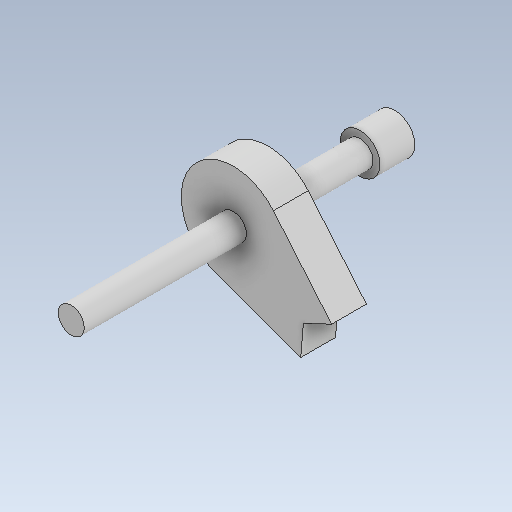
# Autodesk Inventor part: reverser-base
Saved by Autodesk Inventor 2021 (Build 250183000, 183)
## iProperties
Created: 2021-07-09
Part Number: reverser-base
Material: Generic
Document SubType Name: Modeling
Designer: teh18
Density: 1 g/cm^3
Appearance: Default
Author: teh18
Autodesk Inventor part; units mm, degrees
ref_plane "YZ Plane" through (0, 0, 0) normal (1, 0, 0) x (0, 1, 0)
ref_plane "XZ Plane" through (0, 0, 0) normal (0, 1, 0) x (-1, 0, 0)
ref_plane "XY Plane" through (0, 0, 0) normal (0, 0, 1) x (1, 0, 0)
sketch "Sketch1" plane through (0, 0, 0) normal (0, 0, 1) x (1, 0, 0)
  line L0 (3, -1) -> (-3, -1) projected
  line L1 (-3, -1) -> (-3, 1) projected
  line L2 (-3, 1) -> (3, 1) projected
  line L3 (3, 1) -> (3, -1) projected
  circle A0 centre (0, 0) radius 3.75 projected
  line L4 (-3.1, 1.1) -> (-3.1, -1.1)
  line L5 (-3.1, -1.1) -> (3.1, -1.1)
  line L6 (3.1, -1.1) -> (3.1, 1.1)
  line L7 (3.1, 1.1) -> (-3.1, 1.1)
  circle A1 centre (0, 0) radius 5.75
  dimension "d0" = 0.1
  dimension "d5" = 2
  constraints: 8 end point, 1 centre point, 3 other
  measures "d0" distance between parallel lines of L1 L4
  measures "d5" radial gap between concentric circles of A0 A1
extrude "Extrusion1" add sketch "Sketch1" along normal blind 10 contours A0 | A1
sketch "Sketch2" plane through (0, 0, 10) normal (0, 0, 1) x (0, -1, 0)
  line L0 (-1.1, -3.1) -> (-1.1, 3.1) projected
  line L1 (-1.1, 3.1) -> (1.1, 3.1) projected
  line L2 (1.1, 3.1) -> (1.1, -3.1) projected
  line L3 (1.1, -3.1) -> (-1.1, -3.1) projected
  circle A0 centre (0, 0) radius 3.75
  constraints: 1 centre point, 2 other
ref_plane "Work Plane1" through (-14, -11, 93) normal (0, 0, -1) x (0, 1, 0)
extrude "Extrusion2" add sketch "Sketch2" along normal up to surface (83 mm away) contours L0 L1 L2 L3 | A0
ref_plane "Work Plane2" through (0, 0, 36.375) normal (0, 0, -1) x (-1, 0, 0)
sketch "Sketch3" plane through (0, 0, 36.375) normal (0, 0, -1) x (-1, 0, 0)
  circle A0 centre (0, 0) radius 15
  arc A1 (-91.9148, -71.9535) -> (-91.7708, -72.0943) centre (-67.3725, -47) ccw projected
  arc A2 (-99.8859, -53.9357) -> (-101.7483, -40.4192) centre (-102.3703, -47.3915) ccw projected
  arc A3 (-60.0244, -81.22) -> (-73.5792, -79.6604) centre (-66.981, -81.9978) ccw projected
  circle A4 centre (0, 0) radius 30
  line L0 (0, 0) -> (-28.2086, -10.2115)
  line L1 (0, 0) -> (30, 0) construction
  line L2 (0, 0) -> (-19.3236, -22.9477)
  line L3 (0, 0) -> (30, 0) construction
  line L4 (0, 0) -> (-20.0895, -14.0147)
  line L5 (0, 0) -> (25, 0) construction
  line L6 (-19.3236, -22.9477) -> (-20.0895, -14.0147)
  line L7 (-20.0895, -14.0147) -> (-28.2086, -10.2115)
  line L8 (-19.3236, -22.9477) -> (5.1057, -14.1043)
  line L9 (-28.2086, -10.2115) -> (-11.4738, 9.6618)
  arc A5 (-75.9549, -80.9315) -> (-73.5792, -79.6604) centre (-75.4644, -78.9925) ccw projected
  arc A6 (-60.0244, -81.22) -> (-56.998, -80.4271) centre (-67.3725, -47) ccw projected
  line L10 (-56.998, -80.4271) -> (-59.9621, -70.8765) projected
  arc A7 (-59.9621, -70.8765) -> (-52.3252, -27.0356) centre (-67.3725, -47) ccw projected
  line L11 (-52.3252, -27.0356) -> (-43.825, -21.1057) projected
  arc A8 (-76.15, -80.8815) -> (-75.9549, -80.9315) centre (-67.3725, -47) ccw projected
  arc A9 (-99.8859, -53.9357) -> (-101.1035, -56.3392) centre (-99.176, -55.8055) ccw projected
  arc A10 (-101.0492, -56.5332) -> (-98.7606, -57.955) centre (-99.1248, -55.9884) ccw projected
  arc A11 (-92.062, -69.2632) -> (-98.7606, -57.955) centre (-97.4858, -64.8379) ccw projected
  arc A12 (-92.062, -69.2632) -> (-91.9148, -71.9535) centre (-90.5124, -70.5276) ccw projected
  arc A13 (-91.7708, -72.0943) -> (-89.0779, -72.1813) centre (-90.3766, -70.6604) ccw projected
  arc A14 (-77.6226, -78.6253) -> (-89.0779, -72.1813) centre (-84.5324, -77.5047) ccw projected
  arc A15 (-77.6226, -78.6253) -> (-76.15, -80.8815) centre (-75.6484, -78.9454) ccw projected
  circle A16 centre (-67.3725, -47) radius 18 projected
  circle A17 centre (-67.3725, -47) radius 18 projected
  line L12 (-87.3977, -18.2947) -> (-93.1192, -10.0932) projected
  arc A18 (-93.1192, -10.0932) -> (-111.0378, -36.1215) centre (-67.3725, -47) ccw projected
  line L13 (-111.0378, -36.1215) -> (-101.3344, -38.5389) projected
  arc A19 (-101.3344, -38.5389) -> (-101.7483, -40.4192) centre (-67.3725, -47) ccw projected
  arc A20 (-43.825, -21.1057) -> (-87.3977, -18.2947) centre (-67.3725, -47) ccw projected
  arc A21 (-101.1035, -56.3392) -> (-101.0492, -56.5332) centre (-67.3725, -47) ccw projected
  point P0 (-85.3708, -47.2511)
  point P1 (-67.1214, -64.9982)
  point P2 (-67.3725, -47)
  point P3 (-99.176, -55.8055)
  point P4 (-99.1248, -55.9884)
  dimension "d6" = 30
  dimension "d9" = 60
  dimension "d17" = 15
  dimension "d18" = 15
  dimension "d19" = 120
  constraints: 20 end point, 4 point on circle, 3 horizontal, 2 centre point, 2 coincident, 2 equal length, 2 tangent, 1 line through centre
  measures "d6" diameter of A0
  measures "d9" diameter of A4
  measures "d17" angle of L4 L2
  measures "d18" angle of L0 L4
  measures "d19" angle of L7 L6
extrude "Extrusion3" add sketch "Sketch3" against normal blind 10 contours A0 L2 L0 | A0 L0 L9 | L8 L2 A0 | L0 L4 A0 | A0 L4 L7 L0 | L2 L6 L4 A0 | A0 L4 L2
body "Solid1"
